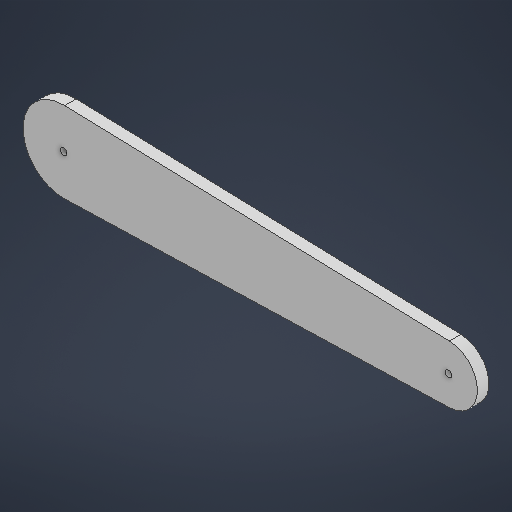
# Autodesk Inventor part: Tibia
Saved by Autodesk Inventor 2026.2 (Build 302298010, 298A)
## iProperties
Created: 2026-07-24
Part Number: Tibia
Material: Generic
Document SubType Name: Modeling
Designer: Entity
Mass: 49.3809 g
Surface Area: 196.719 cm^2
Volume: 49.3809 cm^3
Density: 1 g/cm^3
Appearance: Default
Author: Entity
Autodesk Inventor part; units mm, degrees
ref_plane "YZ Plane" through (0, 0, 0) normal (1, 0, 0) x (0, 1, 0)
ref_plane "XZ Plane" through (0, 0, 0) normal (0, 1, 0) x (-1, 0, 0)
ref_plane "XY Plane" through (0, 0, 0) normal (0, 0, 1) x (1, 0, 0)
sketch "Sketch1" plane through (0, 0, 0) normal (0, 0, 1) x (1, 0, 0)
  circle A0 centre (0, 0) radius 21
  circle A1 centre (200, 0) radius 15
  line L0 (0, 0) -> (200, 0)
  line L1 (0.6307, 20.9905) -> (200.45, 14.9932)
  line L2 (0.6307, -20.9905) -> (200.45, -14.9932)
  dimension "d10" = 15
  dimension "d11" = 21
  dimension "d9" = 200
  constraints: 6 end point, 2 symmetric about line, 1 coincident, 1 horizontal, 7 other
  measures "d9" distance of L0.start L0.end
extrude "Extrusion1" add sketch "Sketch1" along normal blind 6
sketch "Sketch2" plane through (0, 0, 6) normal (0, 0, 1) x (1, 0, 0)
  circle A0 centre (0, 0) radius 1.75
  arc A1 (200.45, -14.9932) -> (200.45, 14.9932) centre (200, 0) ccw projected
  circle A2 centre (200, 0) radius 1.75
  point P0 (293.3543, -13.4475)
  point P1 (293.3543, 13.4475)
  point P2 (250.3596, -14.9957)
  point P3 (250.3596, 14.9957)
  dimension "d5" = 3.5
  dimension "d6" = 3.5
  constraints: 2 centre point, 2 coincident, 1 other
  measures "d5" diameter of A0
  measures "d6" diameter of A2
extrude "Extrusion2" cut sketch "Sketch2" against normal through all
body "Solid1"
